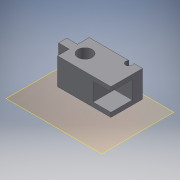
# Autodesk Inventor part: short selector
Saved by Autodesk Inventor 2017 (Build 210142000, 142)
## iProperties
Created: 2018-04-17
Part Number: short selector
Material: Generic
Document SubType Name: Modeling
Designer: RKL
Density: 1 g/cm^3
Appearance: Default
Author: RKL
Autodesk Inventor part; units mm, degrees
ref_plane "YZ Plane" through (0, 0, 0) normal (1, 0, 0) x (0, 1, 0)
ref_plane "XZ Plane" through (0, 0, 0) normal (0, 1, 0) x (-1, 0, 0)
ref_plane "XY Plane" through (0, 0, 0) normal (0, 0, 1) x (1, 0, 0)
ref_plane "Work Plane1" through (0, 0, 0) normal (0, 0, 1) x (1, 0, 0)
sketch "Sketch1" plane through (0, 0, 0) normal (0, 0, 1) x (1, 0, 0)
  circle A0 centre (7, -8.8957) radius 4 construction
  circle A1 centre (-2.136, 8.8957) radius 4 projected
  line L0 (-8.905, 18.405) -> (-8.905, 11.3957) construction
  line L1 (-8.905, 11.3957) -> (-14.905, 11.3957) construction
  line L2 (-14.905, 11.3957) -> (-14.905, 6.3957) construction
  line L3 (-14.905, 6.3957) -> (-8.905, 6.3957) construction
  line L4 (-8.905, 6.3957) -> (-8.905, -6.3957) construction
  line L5 (-8.905, -6.3957) -> (-14.905, -6.3957) construction
  line L6 (-14.905, -6.3957) -> (-14.905, -11.3957) construction
  line L7 (-14.905, -11.3957) -> (-8.905, -11.3957) construction
  line L8 (-8.905, -11.3957) -> (-8.905, -18.405) construction
  line L9 (-8.905, -18.405) -> (15, -18.405) construction
  circle A2 centre (15, -16.5) radius 1.905 construction
  line L10 (15, -18.405) -> (34, -18.405) construction
  line L11 (34, 18.405) -> (34, -18.405) construction
  line L12 (34, 18.405) -> (15, 18.405) construction
  circle A3 centre (15, 16.5) radius 1.905 construction
  line L13 (15, 18.405) -> (-8.905, 18.405) construction
  line L14 (-8.705, 6.5957) -> (-14.705, 6.5957)
  line L15 (-14.705, 6.5957) -> (-14.705, 11.1957)
  line L16 (-14.705, 11.1957) -> (-8.705, 11.1957)
  line L17 (-8.705, 11.1957) -> (-8.705, 6.5957)
  line L18 (-8.705, 0) -> (21.295, 0)
  line L19 (21.295, 0) -> (21.295, 17.7914)
  line L20 (21.295, 17.7914) -> (-8.705, 17.7914)
  line L21 (-8.705, 17.7914) -> (-8.705, 0)
  point P0 (0, 0)
  point P1 (-8.705, 8.8957)
  point P2 (-8.905, 0)
  dimension "d0" = 0.2
  dimension "d1" = 0.2
  dimension "d2" = 0.2
  dimension "d3" = 0.2
  dimension "d4" = 30
  constraints: 16 end point, 4 parallel, 3 midpoint, 2 horizontal, 2 perpendicular, 1 point on line
  measures "d0" distance between parallel lines of L3 L14
  measures "d1" distance between parallel lines of L1 L16
  measures "d2" distance between parallel lines of L2 L15
  measures "d3" distance between parallel lines of L4 L17
  measures "d4" distance between parallel lines of L21 L19
extrude "Extrusion1" add sketch "Sketch1" along normal blind 15
sketch "Sketch2" plane through (0, 0, 15) normal (0, 0, 1) x (1, 0, 0)
  circle A0 centre (15, 16.5) radius 1.905 projected
  point P0 (0, 0)
extrude "Extrusion2" cut sketch "Sketch2" against normal through all
sketch "Sketch3" plane through (21.295, 0, 0) normal (1, 0, 0) x (0, 0, -1)
  line L0 (0, 0) -> (0, 17.7914) construction
  line L1 (0, 17.7914) -> (-15, 17.7914) construction
  line L2 (-15, 0) -> (-15, 17.7914) construction
  line L3 (0, 0) -> (-15, 0) construction
  line L4 (-2.5, 0) -> (-12.5, 0)
  line L5 (-12.5, 0) -> (-12.5, 12)
  line L6 (-12.5, 12) -> (-2.5, 12)
  line L7 (-2.5, 12) -> (-2.5, 0)
  point P0 (0, 0)
  point P1 (-7.5, 0)
  dimension "d9" = 10
  dimension "d10" = 12
  constraints: 8 end point, 2 midpoint, 2 parallel, 1 horizontal, 1 perpendicular
  measures "d9" distance of L5.end L6.end
  measures "d10" distance of L6.end L4.start
extrude "Extrusion3" cut sketch "Sketch3" against normal blind 10
body "Solid1"
